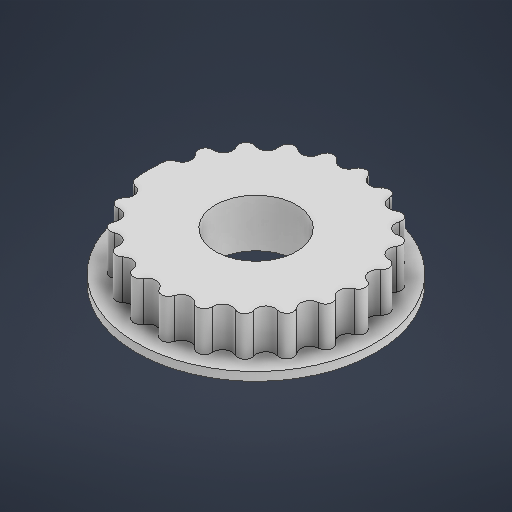
# Autodesk Inventor part: RuedaDentada_v02
Saved by Autodesk Inventor 2026.1 (Build 301233020, 233B)
## iProperties
Created: 2025-10-19
Part Number: RuedaDentada_v02
Material: Generic
Document SubType Name: Modeling
Designer: tito.luyo
Density: 1 g/cm^3
Appearance: Default
Author: tito.luyo
Autodesk Inventor part; units mm, degrees
ref_plane "YZ Plane" through (0, 0, 0) normal (1, 0, 0) x (0, 1, 0)
ref_plane "XZ Plane" through (0, 0, 0) normal (0, 1, 0) x (-1, 0, 0)
ref_plane "XY Plane" through (0, 0, 0) normal (0, 0, 1) x (1, 0, 0)
sketch "Sketch1" plane through (0, 0, 0) normal (0, 1, 0) x (-1, 0, 0)
  line L0 (0, 0) -> (45.711, 0) construction
  line L1 (45.711, 0) -> (45.711, -43.574) construction
  line L2 (45.711, -43.574) -> (0, -43.574) construction
  line L3 (0, -43.574) -> (0, 0) construction
  circle A0 centre (22.5645, -20.681) radius 19.3356
  line L4 (25.3444, -20.681) -> (41.9, -20.681)
  line L5 (22.5645, -20.681) -> (39.1201, -20.681) construction
  circle A1 centre (40.1187, -14.8415) radius 1.65
  line L6 (22.5645, -20.681) -> (40.1187, -14.8415) construction
  line L7 (0, 0) -> (60, 0)
  line L8 (60, 0) -> (60, -60)
  line L9 (60, -60) -> (0, -60)
  line L10 (0, -60) -> (0, 0)
  circle A2 centre (38.0875, -12.7716) radius 1.25
  circle A3 centre (37.6068, -9.9117) radius 1.65
  line L11 (22.5645, -20.681) -> (37.6068, -9.9117) construction
  circle A4 centre (35.0544, -8.535) radius 1.25
  circle A5 centre (33.7495, -5.9452) radius 1.65
  line L12 (22.5645, -20.681) -> (33.7495, -5.9452) construction
  circle A6 centre (30.9042, -5.3848) radius 1.25
  circle A7 centre (26.008, -3.6027) radius 1.25
  line L13 (22.5645, -20.681) -> (28.8918, -3.2966) construction
  circle A8 centre (28.8918, -3.2966) radius 1.65
  circle A9 centre (23.4682, -2.203) radius 1.65
  line L14 (22.5645, -20.681) -> (23.4682, -2.203) construction
  circle A10 centre (20.8039, -3.3482) radius 1.25
  circle A11 centre (15.7572, -4.644) radius 1.25
  line L15 (22.5645, -20.681) -> (17.9637, -2.7622) construction
  circle A12 centre (17.9637, -2.7622) radius 1.65
  line L16 (22.5645, -20.681) -> (12.8707, -4.924) construction
  circle A13 centre (11.4591, -7.4572) radius 1.25
  circle A14 centre (12.8707, -4.924) radius 1.65
  circle A15 centre (5.6639, -13.1563) radius 1.65
  line L17 (22.5645, -20.681) -> (5.6639, -13.1563) construction
  circle A16 centre (5.7681, -16.0545) radius 1.25
  circle A17 centre (5.1511, -21.2282) radius 1.25
  line L18 (22.5645, -20.681) -> (4.1946, -18.4905) construction
  circle A18 centre (4.1946, -18.4905) radius 1.65
  circle A19 centre (8.5057, -30.9704) radius 1.25
  circle A20 centre (6.1697, -29.2519) radius 1.65
  line L19 (22.5645, -20.681) -> (6.1697, -29.2519) construction
  line L20 (22.5645, -20.681) -> (4.3684, -24.0206) construction
  circle A21 centre (6.0917, -26.353) radius 1.25
  circle A22 centre (4.3684, -24.0206) radius 1.65
  circle A23 centre (21.8957, -38.09) radius 1.25
  circle A24 centre (19.0979, -38.8533) radius 1.65
  circle A25 centre (16.7776, -37.1137) radius 1.25
  circle A26 centre (13.8792, -37.0155) radius 1.65
  circle A27 centre (12.1771, -34.6676) radius 1.25
  circle A28 centre (9.4374, -33.7167) radius 1.65
  line L21 (22.5645, -20.681) -> (9.4374, -33.7167) construction
  line L22 (22.5645, -20.681) -> (13.8792, -37.0155) construction
  line L23 (22.5645, -20.681) -> (19.0979, -38.8533) construction
  circle A29 centre (29.9709, -37.6337) radius 1.65
  circle A30 centre (24.6266, -39.0657) radius 1.65
  circle A31 centre (27.0736, -37.5092) radius 1.25
  circle A32 centre (31.8482, -35.4233) radius 1.25
  line L24 (22.5645, -20.681) -> (29.9709, -37.6337) construction
  line L25 (22.5645, -20.681) -> (24.6266, -39.0657) construction
  circle A33 centre (34.6527, -34.6854) radius 1.65
  circle A34 centre (35.7924, -32.0187) radius 1.25
  line L26 (22.5645, -20.681) -> (34.6527, -34.6854) construction
  circle A35 centre (39.726, -22.5987) radius 1.25
  circle A36 centre (40.4507, -25.4067) radius 1.65
  line L27 (22.5645, -20.681) -> (40.4507, -25.4067) construction
  circle A37 centre (38.5535, -27.6) radius 1.25
  circle A38 centre (38.2533, -30.4845) radius 1.65
  line L28 (22.5645, -20.681) -> (38.2533, -30.4845) construction
  circle A39 centre (7.8071, -11.2027) radius 1.25
  circle A40 centre (8.7363, -8.4556) radius 1.65
  line L29 (22.656, -20.6414) -> (8.7363, -8.4556) construction
  circle A41 centre (22.656, -20.6414) radius 7.15
  circle A42 centre (41.0422, -20.0146) radius 1.65
  line L30 (22.5584, -20.7893) -> (41.0422, -20.0146) construction
  circle A43 centre (41.0739, -20.2573) radius 1.65
  line L31 (22.578, -20.6448) -> (41.0739, -20.2573) construction
  circle A44 centre (39.6889, -17.7094) radius 1.25
  arc A45 (40.9575, -22.813) -> (40.9265, -17.5337) centre (16.1823, -20.3187) ccw
  point P0 (40.0384, -23.8091)
  point P1 (41.7675, -22.9405)
  point P2 (38.963, -13.6638)
  point P3 (37.8803, -11.5389)
  point P4 (36.1546, -9.1284)
  point P5 (34.492, -7.4187)
  point P6 (32.1306, -5.6263)
  point P7 (30.0368, -4.4847)
  point P8 (27.251, -3.4708)
  point P9 (24.9133, -2.9994)
  point P10 (21.9523, -2.8546)
  point P11 (19.5797, -3.0956)
  point P12 (16.7083, -3.8329)
  point P13 (14.513, -4.7647)
  point P14 (12.0675, -6.3653)
  point P15 (10.2855, -7.8876)
  point P16 (8.2076, -10.0186)
  point P17 (6.8833, -12.0448)
  point P18 (5.7231, -14.8053)
  point P19 (5.0898, -17.1045)
  point P20 (4.7388, -20.0481)
  point P21 (4.8137, -22.4318)
  point P22 (5.3489, -25.3476)
  point P23 (6.1253, -27.6025)
  point P24 (7.4988, -30.2297)
  point P25 (8.9073, -32.1542)
  point P26 (10.9962, -34.2577)
  point P27 (12.9108, -35.6796)
  point P28 (15.5283, -37.0714)
  point P29 (17.7777, -37.8635)
  point P30 (20.6897, -38.419)
  point P31 (23.0728, -38.5106)
  point P32 (26.0189, -38.1801)
  point P33 (28.3224, -37.5629)
  point P34 (31.039, -36.376)
  point P35 (33.057, -35.1052)
  point P36 (35.3012, -33.1681)
  point P37 (36.8532, -31.3574)
  point P38 (38.4241, -28.8433)
  point P39 (39.3713, -26.6546)
  point P40 (32.7216, -37.1338)
  point P41 (33.0702, -36.9135)
  point P42 (41.5769, -24.2009)
  point P43 (40.8343, -27.0115)
  point P44 (39.6858, -29.6656)
  point P45 (38.1453, -32.1309)
  point P46 (37.439, -33.0346)
  point P47 (36.9604, -33.5892)
  point P48 (41.3184, -15.9742)
  point P49 (40.4008, -13.2157)
  point P50 (36.2633, -34.3267)
  point P51 (34.0627, -36.2262)
  point P52 (39.0879, -10.639)
  point P53 (37.3956, -8.2753)
  point P54 (37.7872, -11.4567)
  point P55 (31.6155, -37.7673)
  point P56 (28.9516, -38.9311)
  point P57 (35.3794, -6.202)
  point P58 (33.0639, -4.4444)
  point P59 (35.1203, -7.0572)
  point P60 (26.1581, -39.6796)
  point P61 (23.2692, -40.0037)
  point P62 (30.5248, -3.06)
  point P63 (27.793, -2.0657)
  point P64 (30.5301, -3.9536)
  point P65 (20.3794, -39.8927)
  point P66 (17.5238, -39.3479)
  point P67 (24.9581, -1.4941)
  point P68 (22.0545, -1.3521)
  point P69 (25.2274, -2.3462)
  point P70 (14.796, -38.3873)
  point P71 (12.2292, -37.0226)
  point P72 (19.1774, -1.6444)
  point P73 (16.3616, -2.3673)
  point P74 (19.6866, -2.3787)
  point P75 (9.9075, -35.2983)
  point P76 (7.8591, -33.2355)
  point P77 (13.6996, -3.4973)
  point P78 (11.2235, -5.0206)
  point P79 (14.4032, -4.0482)
  point P80 (6.1511, -30.9018)
  point P81 (4.8043, -28.3256)
  point P82 (9.0644, -6.8386)
  point P83 (7.1717, -8.9794)
  point P84 (3.8627, -25.5912)
  point P85 (3.338, -22.7319)
  point P86 (6.531, -9.8739)
  point P87 (6.1331, -10.489)
  point P88 (3.2475, -21.5281)
  point P89 (3.2338, -21.1159)
  point P90 (5.5417, -11.5109)
  point P91 (4.3593, -14.1666)
  point P92 (3.2471, -19.8413)
  point P93 (3.5913, -16.9547)
  point P94 (3.8954, -15.6479)
  point P95 (3.7863, -16.0717)
  point P96 (4.445, -16.7734)
  point P97 (4.0998, -22.3062)
  point P98 (8.2473, -32.4539)
  point P99 (6.2223, -27.7264)
  point P100 (13.0608, -35.727)
  point P101 (17.935, -37.8645)
  point P102 (28.4528, -37.4748)
  point P103 (37.17, -31.6384)
  point P104 (39.3832, -26.4978)
  point P105 (39.8742, -16.4732)
  point P106 (39.7762, -18.9564)
  point P107 (39.4265, -20.3492)
  point P108 (39.8411, -21.354)
  point P109 (41.781, -18.5393)
  point P110 (40.7352, -18.3934)
  point P111 (40.9349, -17.6095)
  point P112 (40.9757, -22.6247)
  dimension "d274" = 2.5
  dimension "d315" = 2.5
  dimension "d39" = 0
  dimension "circ_mayor" = 3.3
  dimension "d126" = 18.5
  dimension "d132" = 18.4
  dimension "d133" = 60
  dimension "d134" = 60
  dimension "pos_circ_y" = 22.5645
  dimension "pos_circ_x" = 20.681
  dimension "circ_menor" = 2.5
  dimension "d157" = 3.3
  dimension "d158" = 18.5
  dimension "d160" = 2.5
  dimension "d166" = 17.2
  dimension "d167" = 3.3
  dimension "d168" = 18.5
  dimension "d169" = 2.5
  dimension "d170" = 3.3
  dimension "d171" = 18.5
  dimension "d172" = 2.5
  dimension "d173" = 17.2
  dimension "d177" = 17.2
  dimension "d178" = 3.3
  dimension "d179" = 18.5
  dimension "d180" = 2.5
  dimension "d181" = 3.3
  dimension "d182" = 18.5
  dimension "d183" = 2.5
  dimension "d184" = 17.2
  dimension "d185" = 3.3
  dimension "d186" = 18.5
  dimension "d187" = 2.5
  dimension "d192" = 17.2
  dimension "d196" = 17.2
  dimension "d197" = 3.3
  dimension "d198" = 18.5
  dimension "d199" = 2.5
  dimension "d200" = 3.3
  dimension "d201" = 18.5
  dimension "d202" = 2.5
  dimension "d203" = 17.2
  dimension "d204" = 3.3
  dimension "d205" = 18.5
  dimension "d206" = 2.5
  dimension "d207" = 3.3
  dimension "d208" = 18.5
  dimension "d209" = 2.5
  dimension "d210" = 17.2
  dimension "d211" = 17.2
  dimension "d212" = 3.3
  dimension "d213" = 18.5
  dimension "d214" = 2.5
  dimension "d215" = 3.3
  dimension "d216" = 18.5
  dimension "d217" = 2.5
  dimension "d218" = 17.2
  dimension "d219" = 3.3
  dimension "d220" = 18.5
  dimension "d221" = 2.5
  dimension "d226" = 17.2
  dimension "d227" = 17.2
  dimension "d253" = 3.3
  dimension "d254" = 18.5
  dimension "d255" = 2.5
  dimension "d256" = 3.3
  constraints: 56 end point, 43 centre point, 38 tangent, 3 coincident, 2 horizontal, 2 parallel, 2 point on circle, 1 collinear, 1 perpendicular, 15 other
  measures "d39" distance between parallel lines of L4 L5
  measures "circ_mayor" diameter of A1
  measures "d126" distance of L5.start L6.end
  measures "d132" angle of L4 L6
  measures "d133" distance of L8.end L9.end
  measures "d134" distance of L7.end L8.end
  measures "pos_circ_y" distance from line of L10 point (22.564, -20.681)
  measures "pos_circ_x" distance from line of L7 point (22.564, -20.681)
  measures "circ_menor" diameter of A2
  measures "d157" diameter of A3
  measures "d158" distance of L5.start L11.end
  measures "d160" diameter of A4
  measures "d166" angle of L6 L11
  measures "d167" diameter of A5
  measures "d168" distance of L5.start L12.end
  measures "d169" diameter of A6
  measures "d170" diameter of A8
  measures "d171" distance of L5.start L13.end
  measures "d172" diameter of A7
  measures "d173" angle of L12 L13
  measures "d177" angle of L11 L12
  measures "d178" diameter of A9
  measures "d179" distance of L5.start L14.end
  measures "d180" diameter of A10
  measures "d181" diameter of A12
  measures "d182" distance of L5.start L15.end
  measures "d183" diameter of A11
  measures "d184" angle of L14 L15
  measures "d185" diameter of A14
  measures "d186" distance of L5.start L16.end
  measures "d187" diameter of A13
  measures "d192" angle of L15 L16
  measures "d196" angle of L13 L14
  measures "d197" diameter of A15
  measures "d198" distance of L5.start L17.end
  measures "d199" diameter of A16
  measures "d200" diameter of A18
  measures "d201" distance of L5.start L18.end
  measures "d202" diameter of A17
  measures "d203" angle of L17 L18
  measures "d204" diameter of A22
  measures "d205" distance of L5.start L20.end
  measures "d206" diameter of A21
  measures "d207" diameter of A20
  measures "d208" distance of L5.start L19.end
  measures "d209" diameter of A19
  measures "d210" angle of L20 L19
  measures "d211" angle of L18 L20
  measures "d212" diameter of A28
  measures "d213" distance of L5.start L21.end
  measures "d214" diameter of A27
  measures "d215" diameter of A26
  measures "d216" distance of L5.start L22.end
  measures "d217" diameter of A25
  measures "d218" angle of L21 L22
  measures "d219" diameter of A24
  measures "d220" distance of L5.start L23.end
  measures "d221" diameter of A23
  measures "d226" angle of L22 L23
  measures "d227" angle of L19 L21
  measures "d253" diameter of A30
  measures "d254" distance of L5.start L25.end
  measures "d255" diameter of A31
  measures "d256" diameter of A29
extrude "Extrusion1" add sketch "Sketch1" along normal blind 7 contours A45 A42 L4 | L4 A42 A43 A45 | A45 A42 A44 | A43 A44 A42 A45 | A45 A43 A35 A42 | A42 A35 A43 L4 | L4 A43 A42 | A43 A42 A44 | A44 A42 | A45 A35 A43 | A35 A43 | A43 A35 A36 A37 A38 A34 A33 A32 A29 A31 A30 A23 A24 A25 A26 A27 A28 A19 A20 A21 A22 A17 A18 A16 A15 A39 A40 A13 A14 A11 A12 A10 A9 A7 A8 A6 A5 A4 A3 A2 A1 A44 A42 | A44 A42 | A35 A43 | A2 | A37 | A4 | A34 | A6 | A32 | A7 | A31 | A10 | A23 | A11 | A25 | A13 | A27 | A39 | A19 | A16 | A21 | A17
sketch "Sketch2" plane through (0, 0, 0) normal (0, -1, 0) x (1, 0, 0)
  circle A0 centre (-22.656, -20.6414) radius 7.15 projected
  circle A1 centre (-22.656, -20.6414) radius 21.1114
  point P0 (0, 0)
  constraints: 1 centre point, 1 coincident
extrude "Extrusion2" add sketch "Sketch2" along normal blind 1.5
equation "\"angulo\" = 17.2deg"
equation "\"sep\" = 18.5"
equation "\"d144\" = 18.5"
equation "\"d148\" = 18.5"
equation "\"d162\" = 18.5"
equation "\"d163\" = 18.5"
equation "\"d164\" = 17.2deg"
equation "\"d174\" = 18.5"
equation "\"d175\" = 17.2deg"
equation "\"d193\" = 18.5"
equation "\"d194\" = 17.2deg"
equation "\"d228\" = 18.5"
equation "\"d229\" = 17.2deg"
equation "\"d247\" = 18.5"
equation "\"d250\" = 17.2deg"
equation "\"d261\" = 18.5"
equation "\"d263\" = 17.2deg"
equation "\"d278\" = 18.5"
equation "\"d280\" = 17.2deg"
equation "\"d281\" = 17.2deg"
equation "\"d289\" = 18.5"
equation "\"d310\" = 18.5"
equation "\"d316\" = 18.5"
body "Solid1"
